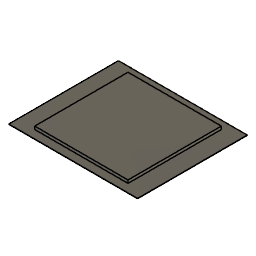
proiect_tsc-pcb3D (Autodesk Fusion 360 archive; units mm, degrees)
design "piesa-proect-epaper-final"
part number: 2026-03-29-15-02-46-541
Autodesk Fusion 360 part; units mm, degrees
sketch "Sketch1" plane through (0, 0, 0) normal (0, 0, 1) x (1, 0, 0)
  line L0 (18.66, 15.9) -> (-18.66, 15.9)
  line L1 (-18.66, 15.9) -> (-18.66, -15.9)
  line L2 (-18.66, -15.9) -> (18.66, -15.9)
  line L3 (18.66, -15.9) -> (18.66, 15.9)
  line L4 (18.66, 15.9) -> (-18.66, -15.9) construction
  line L5 (-18.66, 15.9) -> (18.66, -15.9) construction
  dimension "d1" = 37.32
  dimension "d2" = 31.8
  constraint horizontal L0
  constraint perpendicular L0 L1
  constraint parallel L0 L2
  constraint parallel L1 L3
  constraint coincident L4 origin
  constraint coincident L5 origin
  measures "d1" distance of L1.end L2.end
  measures "d2" distance of L0.end L1.end
extrude "Extrude1" add sketch "Sketch1" along normal blind 0.1
sketch "Sketch2" plane through (0, 0, 0) normal (0, 0, 1) x (1, 0, 0)
  line L0 (13.5, -13.5) -> (-13.5, -13.5)
  line L1 (-13.5, -13.5) -> (-13.5, 13.5)
  line L2 (-13.5, 13.5) -> (13.5, 13.5)
  line L3 (13.5, 13.5) -> (13.5, -13.5)
  line L4 (13.5, -13.5) -> (-13.5, 13.5) construction
  line L5 (-13.5, -13.5) -> (13.5, 13.5) construction
  dimension "d5" = 27
  dimension "d6" = 27
  constraint horizontal L0
  constraint perpendicular L0 L1
  constraint parallel L0 L2
  constraint parallel L1 L3
  constraint coincident L4 origin
  constraint coincident L5 origin
  measures "d5" distance of L1.end L2.end
  measures "d6" distance of L0.end L1.end
extrude "Extrude2" add sketch "Sketch2" along normal blind 0.95

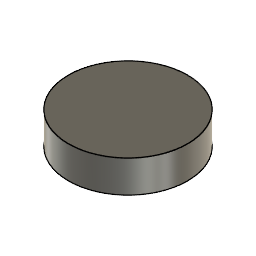
design "shaker-piesa-proiect"
part number: 2026-03-29-14-57-19-738
Autodesk Fusion 360 part; units mm, degrees
sketch "Sketch1" plane through (0, 0, 0) normal (0, 0, 1) x (1, 0, 0)
  circle A0 centre (0, 0) radius 5
  dimension "d1" = 10
  constraint coincident A0.centre origin
  measures "d1" diameter of A0
extrude "Extrude1" add sketch "Sketch1" along normal blind 2.7
